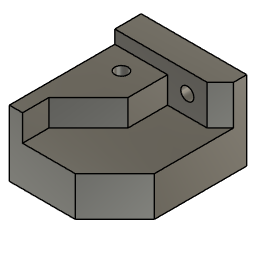
Robocon_Task1C_1 (Autodesk Fusion 360 design; units mm, degrees)
Autodesk Fusion 360 part; units mm, degrees
sketch "Sketch1" plane through (0, 0, 0) normal (0, 0, 1) x (1, 0, 0) in component "Component"
  line L0 (80, -100) -> (-80, -100)
  line L1 (-80, -100) -> (-80, 100)
  line L2 (-80, 100) -> (80, 100)
  line L3 (80, 100) -> (80, -100)
  line L4 (80, -100) -> (-80, 100) construction
  line L5 (-80, -100) -> (80, 100) construction
  dimension "d1" = 160
  dimension "d2" = 200
  constraint horizontal L0
  constraint perpendicular L0 L1
  constraint parallel L0 L2
  constraint parallel L1 L3
  constraint coincident L4 origin
  constraint coincident L5 origin
  measures "d1" distance of L1.end L2.end
  measures "d2" distance of L0 L2
extrude "Extrude1" add sketch "Sketch1" along normal blind 60 in component "Component"
sketch "Sketch5" plane through (0, 0, 60) normal (0, 0, 1) x (-1, 0, 0) in component "Component"
  line L0 (-80, -100) -> (80, -100)
  line L1 (80, -100) -> (80, 100)
  line L2 (80, 100) -> (-80, 100)
  line L3 (-80, 100) -> (-80, -100)
  line L4 (-20, 100) -> (-80, 40)
  constraint coincident L2 L4.start
  constraint coincident L3 L4.end
extrude "Extrude3" cut sketch "Sketch5" against normal up to surface (60 mm away) contours L2 L3 L4 in component "Component"
sketch "Sketch6" plane through (0, 0, 60) normal (0, 0, 1) x (-1, 0, 0) in component "Component"
  line L0 (-20, 100) -> (-80, 40)
  line L1 (-80, 40) -> (-80, -100)
  line L2 (-80, -100) -> (80, -100)
  line L3 (80, -100) -> (80, 100)
  line L4 (80, 100) -> (-20, 100)
  line L5 (60, 100) -> (60, 60)
  line L6 (60, 60) -> (0, 0)
  line L7 (0, 0) -> (0, -60)
  line L8 (0, -60) -> (80, -60)
  line L9 (80, 100) -> (60, 100)
  constraint coincident L4 L5.start
  constraint perpendicular L4 L5
  constraint coincident L6.end L7.start
  constraint parallel L0 L6
  constraint perpendicular L4 L7
  constraint coincident L3 L8.end
  constraint perpendicular L3 L8
  constraint coincident L3.end L4.start
extrude "Extrude4" add sketch "Sketch6" along normal blind 40 contours L3 L4 L5 L6 L7 L8 L9 in component "Component"
sketch "Sketch7" plane through (0, 0, 60) normal (0, 0, 1) x (-1, 0, 0) in component "Component"
  line L0 (60, 60) -> (60, 100)
  line L1 (60, 100) -> (-20, 100)
  line L2 (-20, 100) -> (-80, 40)
  line L3 (-80, 40) -> (-80, -100)
  line L4 (-80, -100) -> (80, -100)
  line L5 (80, -100) -> (80, -60)
  line L6 (80, -60) -> (0, -60)
  line L7 (0, -60) -> (0, 0)
  line L8 (0, 0) -> (60, 60)
  line L9 (-60, -60) -> (-80, -80)
  line L10 (-80, -100) -> (80, -100)
  line L11 (80, -60) -> (-60, -60)
  constraint coincident L3 L9.end
  constraint coincident L3.end L4.start
  constraint coincident L4.end L5.start
  constraint coincident L5.end L6.start
  constraint perpendicular L7 L11
extrude "Extrude5" add sketch "Sketch7" along normal blind 60 contours L3 L4 L5 L6 L9 L10 L11 in component "Component"
sketch "Sketch8" plane through (0, 0, 100) normal (0, 0, 1) x (-1, 0, 0) in component "Component"
  line L0 (80, 100) -> (60, 100)
  line L1 (60, 100) -> (60, 60)
  line L2 (60, 60) -> (0, 0)
  line L3 (0, 0) -> (0, -60)
  line L4 (0, -60) -> (80, -60)
  line L5 (80, -60) -> (80, 100)
  circle A0 centre (40, -30) radius 10
  dimension "d14" = 40
  dimension "d15" = 30
  dimension "d16" = 20
  measures "d14" distance of L5 A0.centre
  measures "d15" distance of L4 A0.centre
  measures "d16" diameter of A0
extrude "Extrude6" cut sketch "Sketch8" against normal up to surface (100 mm away) contours A0 in component "Component"
sketch "Sketch9" plane through (0, 60, 0) normal (0, -1, 0) x (1, 0, 0) in component "Component"
  line L0 (-80, 100) -> (0, 100)
  line L1 (0, 100) -> (0, 60)
  line L2 (0, 60) -> (60, 60)
  line L3 (60, 60) -> (60, 120)
  line L4 (60, 120) -> (-80, 120)
  line L5 (-80, 120) -> (-80, 100)
  circle A0 centre (30, 90) radius 10
  dimension "d19" = 30
  dimension "d20" = 30
  dimension "d21" = 20
  measures "d19" distance of L4 A0.centre
  measures "d20" distance of L3 A0.centre
  measures "d21" diameter of A0
extrude "Extrude7" cut sketch "Sketch9" against normal up to surface (40 mm away) contours A0 in component "Component"
component "Component" placed x (1, 0, 0) y (0, 1, 0) z (0, 0, 1) at (0, 0, 0)
